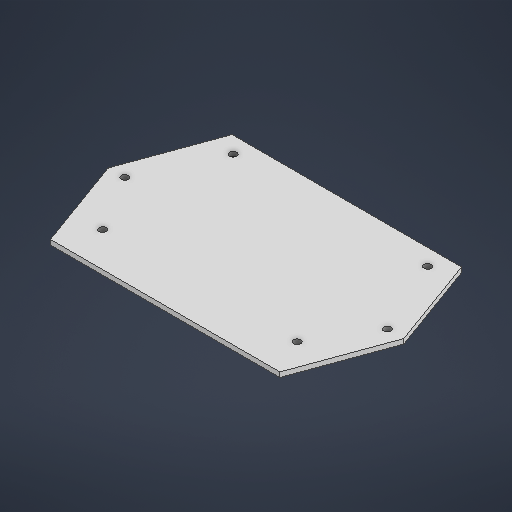
# Autodesk Inventor part: ControllerHeadBottom
Saved by Autodesk Inventor 2026.2 (Build 302298010, 298A)
## iProperties
Created: 2026-03-18
Part Number: ControllerHeadBottom
Material: Generic
Document SubType Name: Modeling
Designer: barbe
Density: 1 g/cm^3
Appearance: Default
Author: barbe
Autodesk Inventor part; units mm, degrees
ref_plane "YZ Plane" through (0, 0, 0) normal (1, 0, 0) x (0, 1, 0)
ref_plane "XZ Plane" through (0, 0, 0) normal (0, 1, 0) x (-1, 0, 0)
ref_plane "XY Plane" through (0, 0, 0) normal (0, 0, 1) x (1, 0, 0)
sketch "Sketch1" plane through (0, 0, 0) normal (0, 1, 0) x (-1, 0, 0)
  line L0 (45.72, 36.195) -> (-45.72, 36.195)
  line L1 (-45.72, 36.195) -> (-45.72, -36.195)
  line L2 (-45.72, -36.195) -> (45.72, -36.195)
  line L3 (45.72, -36.195) -> (45.72, 36.195)
  line L4 (45.72, 36.195) -> (-45.72, -36.195) construction
  line L5 (-45.72, 36.195) -> (45.72, -36.195) construction
  line L6 (48, 38) -> (-48, 38)
  line L7 (-48, 38) -> (-48, -38)
  line L8 (-48, -38) -> (48, -38)
  line L9 (48, -38) -> (48, 38)
  line L10 (48, 38) -> (-48, -38) construction
  line L11 (-48, 38) -> (48, -38) construction
  line L12 (-48, 38) -> (-61.8309, 0)
  line L13 (-48, 38) -> (-7.5612, 38) construction
  line L14 (-48, -38) -> (-61.8309, 0)
  line L15 (-48, -38) -> (-7.5612, -38) construction
  line L16 (0, -38) -> (0, 38)
  line L17 (-48, 0) -> (48, 0)
  line L18 (48, 38) -> (61.8309, 0)
  line L19 (48, -38) -> (61.8309, 0)
  circle A0 centre (54.9154, 0) radius 1.5
  circle A1 centre (-54.9154, 0) radius 1.5
  circle A2 centre (40.64, -31.115) radius 1.5
  circle A3 centre (40.64, 23.495) radius 1.5
  circle A4 centre (-40.64, -31.115) radius 1.5
  circle A5 centre (-40.64, 23.495) radius 1.5
  line L20 (61.8309, 0) -> (48, 0)
  line L21 (-48, 0) -> (-61.8309, 0)
  point P0 (0, 0)
  point P1 (0, 0)
  dimension "d43" = 91.44
  dimension "d44" = 72.39
  dimension "d45" = 96
  dimension "d46" = 76
  dimension "d47" = 110
  dimension "d48" = 110
  dimension "d49" = 3
  dimension "d50" = 3
  dimension "d51" = 3
  dimension "d52" = 5.08
  dimension "d53" = 5.08
  dimension "d54" = 3
  dimension "d55" = 12.7
  dimension "d56" = 5.08
  constraints: 44 end point, 9 midpoint, 6 centre point, 4 horizontal, 4 parallel, 3 symmetric about line, 2 equal length, 2 perpendicular, 2 other
  measures "d43" distance of L2.end L1.end
  measures "d44" distance of L1.end L0.end
  measures "d45" distance of L8.end L7.end
  measures "d46" distance of L7.end L6.end
  measures "d47" angle of L12 L13
  measures "d48" angle of L15 L14
  measures "d49" diameter of A0
  measures "d50" diameter of A1
  measures "d51" diameter of A2
  measures "d52" horizontal distance of A2.centre L2.end
  measures "d53" distance from line of L3 A2.centre
  measures "d54" diameter of A3
  measures "d55" distance from line of L0 A3.centre
  measures "d56" distance from line of L3 A3.centre
extrude "Extrusion3" add sketch "Sketch1" along normal blind 2 contours L3 L17 L16 L0 | L0 L16 L6 L9 L17 L3 | L16 L17 L1 L0 | L0 L1 L17 L7 L6 L16 | L17 L9 L8 L16 L2 L3 | L3 L2 L16 L17 | L16 L2 L1 L17 | L20 A0 L19 L9 | L9 L18 L20 A0 | L1 L2 L16 L8 L7 L17 | L7 L21 A1 L12 | L7 L14 L21 A1
thread "Thread7" size "M3x0.5" class "6H" standard "ANSI Metric M Profile" length 8.001
thread "Thread8" size "M3x0.5" class "6H" standard "ANSI Metric M Profile" length 8.001
thread "Thread9" size "M3x0.5" class "6H" standard "ANSI Metric M Profile" length 8.001
thread "Thread10" size "M3x0.5" class "6H" standard "ANSI Metric M Profile" length 8.001
thread "Thread11" size "M3x0.5" class "6H" standard "ANSI Metric M Profile" length 8.001
thread "Thread12" size "M3x0.5" class "6H" standard "ANSI Metric M Profile" length 8.001
body "Solid3"
